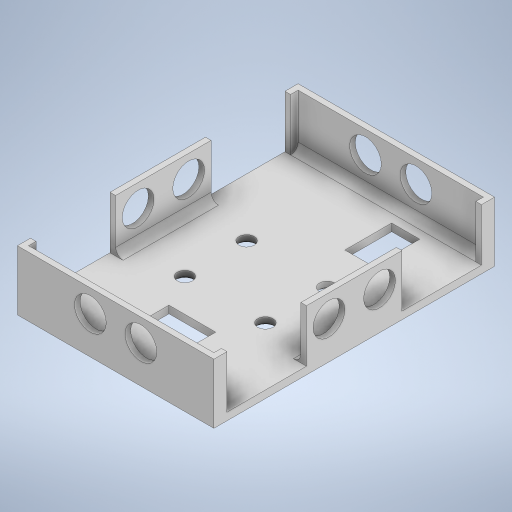
# Autodesk Inventor part: TestingPlatform_base01
Saved by Autodesk Inventor 2024.2 (Build 282272000, 272)
## iProperties
Created: 2024-01-29
Part Number: TestingPlatform_base01
Material: Generic
Document SubType Name: Modeling
Designer: ringl
Density: 1 g/cm^3
Appearance: Default
Author: ringl
Autodesk Inventor part; units mm, degrees
ref_plane "YZ Plane" through (0, 0, 0) normal (1, 0, 0) x (0, 1, 0)
ref_plane "XZ Plane" through (0, 0, 0) normal (0, 1, 0) x (-1, 0, 0)
ref_plane "XY Plane" through (0, 0, 0) normal (0, 0, 1) x (1, 0, 0)
sketch "Sketch1" plane through (0, 0, 0) normal (0, 1, 0) x (-1, 0, 0)
  line L0 (0, 0) -> (58, 0) construction
  line L1 (58, 0) -> (58, -48) construction
  line L2 (58, -48) -> (0, -48) construction
  line L3 (0, -48) -> (0, 0) construction
  circle A0 centre (50.5, -7.5) radius 2.35
  circle A1 centre (50.5, -40.5) radius 2.35
  circle A2 centre (7.5, -7.5) radius 2.35
  circle A3 centre (7.5, -40.5) radius 2.35
  circle A4 centre (50.5, -7.5) radius 5
  circle A5 centre (50.5, -40.5) radius 5
  circle A6 centre (7.5, -7.5) radius 5
  circle A7 centre (7.5, -40.5) radius 5
  dimension "d0" = 58
  dimension "d1" = 48
  dimension "d2" = 4.7
  dimension "d3" = 4.7
  dimension "d4" = 4.7
  dimension "d5" = 4.7
  dimension "d6" = 33
  dimension "d7" = 43
  dimension "d8" = 7.5
  dimension "d9" = 7.5
  dimension "d10" = 7.5
  dimension "d11" = 7.5
  dimension "d12" = 7.5
  dimension "d13" = 7.5
  dimension "d14" = 10
  dimension "d15" = 10
  dimension "d16" = 10
  dimension "d17" = 10
  constraints: 8 centre point, 8 end point, 4 coincident, 2 parallel, 1 horizontal, 1 perpendicular
  measures "d0" distance of L1.end L2.end
  measures "d1" distance of L0.end L1.end
  measures "d2" diameter of A0
  measures "d3" diameter of A1
  measures "d4" diameter of A2
  measures "d5" diameter of A3
  measures "d6" distance of A1.centre A0.centre
  measures "d7" distance of A3.centre A1.centre
  measures "d8" distance from line of L0 A0.centre
  measures "d9" distance from line of L0 A2.centre
  measures "d10" distance from line of L3 A2.centre
  measures "d11" distance from line of L3 A3.centre
  measures "d12" distance from line of L1 A1.centre
  measures "d13" distance from line of L1 A0.centre
  measures "d14" diameter of A4
  measures "d15" diameter of A5
  measures "d16" diameter of A6
  measures "d17" diameter of A7
extrude "Extrusion1" add sketch "Sketch1" along normal blind 12
sketch "Sketch2" plane through (-50.5, 12, -7.5) normal (0, 1, 0) x (1, 0, 0)
  line L0 (-31, -58.5) -> (74, -58.5)
  line L1 (74, -58.5) -> (74, 91.5)
  line L2 (74, 91.5) -> (-31, 91.5)
  line L3 (-31, 91.5) -> (-31, -58.5)
  circle A0 centre (0, 0) radius 2.35 projected
  circle A1 centre (0, 33) radius 2.35 projected
  circle A2 centre (43, 33) radius 2.35 projected
  circle A3 centre (43, 0) radius 2.35 projected
  circle A4 centre (43, 0) radius 2.35
  point P0 (50.5, -7.5)
  dimension "d20" = 105
  dimension "d21" = 150
  dimension "d22" = 58.5
  dimension "d23" = 31
  constraints: 8 end point, 4 coincident, 2 parallel, 1 centre point, 1 horizontal, 1 perpendicular, 1 other
  measures "d20" distance of L2.end L1.end
  measures "d21" distance of L1.end L0.end
  measures "d22" distance from line of L0 point (43, 0)
  measures "d23" distance from line of L3 point (0, 0)
extrude "Extrusion3" add sketch "Sketch2" along normal blind 4
sketch "Sketch3" plane through (-50.5, 16, -7.5) normal (0, 1, 0) x (1, 0, 0)
  line L0 (-31, 91.5) -> (-31, -58.5) projected
  line L1 (-31, -58.5) -> (-31, -38.5)
  line L2 (-31, -38.5) -> (-28, -38.5)
  line L3 (-28, -38.5) -> (-28, -55.5)
  line L4 (-28, -55.5) -> (-11, -55.5)
  line L5 (-11, -58.5) -> (-31, -58.5)
  line L6 (-28, 88.5) -> (-11, 88.5)
  line L7 (74, -58.5) -> (74, 91.5) projected
  line L8 (74, 91.5) -> (54, 91.5)
  line L9 (71, 71.5) -> (74, 71.5)
  line L10 (74, 71.5) -> (74, 91.5)
  line L11 (74, -58.5) -> (74, -38.5)
  line L12 (74, -38.5) -> (71, -38.5)
  line L13 (71, -38.5) -> (71, -55.5)
  line L14 (71, -55.5) -> (54, -55.5)
  line L15 (54, -58.5) -> (74, -58.5)
  line L16 (74, 91.5) -> (-31, 91.5) projected
  line L17 (54, 88.5) -> (71, 88.5)
  line L18 (71, 88.5) -> (71, 71.5)
  line L19 (-11, 91.5) -> (-31, 91.5)
  line L20 (-31, 91.5) -> (-31, 71.5)
  line L21 (-31, 71.5) -> (-28, 71.5)
  line L22 (-28, 71.5) -> (-28, 88.5)
  line L23 (-11, -55.5) -> (54, -55.5)
  line L24 (54, -58.5) -> (-11, -58.5)
  line L25 (-11, 91.5) -> (54, 91.5)
  line L26 (54, 88.5) -> (-11, 88.5)
  point P0 (50.5, -7.5)
  dimension "d28" = 20
  dimension "d48" = 20
  dimension "d49" = 3
  dimension "d50" = 3
  dimension "d51" = 3
  dimension "d52" = 3
  dimension "d53" = 20
  dimension "d55" = 20
  dimension "d56" = 20
  dimension "d57" = 3
  dimension "d69" = 20
  dimension "d95" = 17
  dimension "d96" = 65
  dimension "d102" = 3
  dimension "d103" = 17
  dimension "d104" = 65
  dimension "d105" = 17
  constraints: 48 end point, 10 perpendicular, 6 point on line, 4 collinear, 2 horizontal, 1 parallel
  measures "d28" distance of L0.end L1.end
  measures "d48" distance of L5.start L0.end
  measures "d49" distance of L4.end L5.start
  measures "d50" distance of L1.end L2.end
  measures "d51" distance of L14.end L15.start
  measures "d52" distance of L11.end L12.end
  measures "d53" distance between parallel lines of L15 L12
  measures "d55" distance of L7.end L8.end
  measures "d56" distance of L9.end L7.end
  measures "d57" distance of L9.start L9.end
  measures "d69" distance of L0.start L20.end
  measures "d95" distance of L13.end L14.end
  measures "d96" distance of L4.end L14.end
  measures "d102" distance between parallel lines of L16 L17
  measures "d103" distance of L6.start L6.end
  measures "d104" distance of L17.start L6.end
  measures "d105" distance of L17.start L17.end
extrude "Extrusion4" add sketch "Sketch3" along normal blind 28 contours L16 L8 L7 L9 L18 L17 L26 L6 L22 L21 L0 | L2 L3 L4 L23 L14 L13 L12 L7 L15 L24 L5 L0
sketch "Sketch4" plane through (-81.5, 12, 51) normal (0, 0, 1) x (1, 0, 0)
  line L0 (0, 0) -> (0, 32) projected
  line L1 (0, 0) -> (100, 0)
  line L2 (100, 0) -> (100, -15)
  line L3 (100, -15) -> (0, -15)
  line L4 (0, -15) -> (0, 0)
  point P0 (81.5, -12)
  dimension "d59" = 100
  dimension "d60" = 15
  constraints: 8 end point, 2 parallel, 1 horizontal, 1 perpendicular
  measures "d59" distance of L2.end L3.end
  measures "d60" distance of L1.end L2.end
extrude "remove legs" cut sketch "Sketch4" against normal through all
sketch "Sketch5" plane through (-50.5, 12, -7.5) normal (0, -1, 0) x (1, 0, 0)
  circle A0 centre (0, 0) radius 2.35 projected
  circle A1 centre (0, 0) radius 4.1
  circle A2 centre (43, 0) radius 2.35 projected
  circle A3 centre (43, 0) radius 4.1
  circle A4 centre (43, -33) radius 2.35 projected
  circle A5 centre (43, -33) radius 4.1
  circle A6 centre (0, -33) radius 2.35 projected
  circle A7 centre (0, -33) radius 4.1
  circle A8 centre (0, 0) radius 2.35
  circle A9 centre (43, 0) radius 2.35
  circle A10 centre (43, -33) radius 2.35
  circle A11 centre (0, -33) radius 2.35
  point P0 (50.5, 7.5)
  dimension "d63" = 8.2
  dimension "d64" = 8.2
  dimension "d65" = 8.2
  dimension "d66" = 8.2
  constraints: 8 centre point, 8 coincident, 4 concentric
  measures "d63" diameter of A1
  measures "d64" diameter of A3
  measures "d65" diameter of A5
  measures "d66" diameter of A7
extrude "Extrusion6" cut sketch "Sketch5" against normal blind 4
sketch "Sketch6" plane through (-50.5, 16, -7.5) normal (0, 1, 0) x (1, 0, 0)
  line L0 (9, -17.5) -> (34, -17.5)
  line L1 (34, -17.5) -> (34, -32.5)
  line L2 (34, -32.5) -> (9, -32.5)
  line L3 (9, -32.5) -> (9, -17.5)
  line L4 (30.5, 55) -> (45.5, 55)
  line L5 (45.5, 55) -> (45.5, 80)
  line L6 (45.5, 80) -> (30.5, 80)
  line L7 (30.5, 80) -> (30.5, 55)
  circle A0 centre (43, 33) radius 4.1 construction
  circle A1 centre (0, 33) radius 4.1 construction
  circle A2 centre (0, 0) radius 4.1 construction
  circle A3 centre (43, 0) radius 4.1 construction
  point P0 (50.5, -7.5)
  dimension "d72" = 25
  dimension "d73" = 15
  dimension "d74" = 15
  dimension "d75" = 25
  dimension "d76" = 22
  dimension "d77" = 2.5
  dimension "d78" = 9
  dimension "d79" = 17.5
  constraints: 16 end point, 4 parallel, 2 horizontal, 2 perpendicular
  measures "d72" distance of L0.start L0.end
  measures "d73" distance of L4.start L4.end
  measures "d74" distance of L0.end L1.end
  measures "d75" distance of L4.end L5.end
  measures "d76" distance from line of L4 A0.centre
  measures "d77" distance from line of A0.centre L5
  measures "d78" distance from line of L3 A2.centre
  measures "d79" distance from line of L0 A3.centre
extrude "Extrusion7" cut sketch "Sketch6" against normal blind 10
chamfer "Chamfer1" distance 1 angle 45 4 edges at (-11.6, 12, -7.5) (-11.6, 12, -40.5) (-54.6, 12, -40.5) (-54.6, 12, -7.5)
sketch "Sketch7" plane through (-50.5, 16, -7.5) normal (0, 1, 0) x (1, 0, 0)
  line L0 (74, -38.5) -> (74, 71.5) projected
  line L1 (74, 42) -> (71, 42)
  line L2 (71, 42) -> (71, -9)
  line L3 (71, -9) -> (74, -9)
  line L4 (74, -9) -> (74, 42)
  line L5 (-31, 71.5) -> (-31, -38.5) projected
  line L6 (-31, 42) -> (-28, 42)
  line L7 (-28, 42) -> (-28, -9)
  line L8 (-28, -9) -> (-31, -9)
  line L9 (-31, -9) -> (-31, 42)
  line L10 (-31, -58.5) -> (74, -58.5) projected
  point P0 (50.5, -7.5)
  point P1 (74, -28.5)
  point P2 (74, 61.5)
  point P3 (-31, 67.5)
  point P4 (-31, -28.5)
  point P5 (72.5, 42)
  point P6 (-29.5, 42)
  point P7 (-31, -9)
  point P8 (74, -48.5)
  point P9 (-31, -48.5)
  dimension "d88" = 3
  dimension "d89" = 51
  dimension "d91" = 3
  dimension "d92" = 51
  dimension "d116" = 49.5
  constraints: 16 end point, 4 parallel, 2 horizontal, 2 midpoint, 2 perpendicular, 2 point on line, 1 horizontal alignment
  measures "d88" distance of L1.start L1.end
  measures "d89" distance of L1.end L2.end
  measures "d91" distance of L7.end L8.end
  measures "d92" distance of L6.end L7.end
  measures "d116" distance between parallel lines of L10 L3
sketch "Sketch8" plane through (23.5, 12, 51) normal (1, 0, 0) x (0, 0, -1)
  circle A0 centre (61.5, 20) radius 8.5
  circle A1 centre (88.5, 20) radius 8.5
  line L0 (0, 0) -> (150, 0) projected
  line L1 (0, 0) -> (0, 32) projected
  point P0 (51, -12)
  dimension "d106" = 17
  dimension "d107" = 17
  dimension "d108" = 27
  dimension "d109" = 20
  dimension "d119" = 61.5
  constraints: 2 centre point, 1 horizontal alignment
  measures "d106" diameter of A0
  measures "d107" diameter of A1
  measures "d108" distance of A1.centre A0.centre
  measures "d109" distance from line of L0 A0.centre
  measures "d119" distance from line of L1 A0.centre
sketch "Sketch9" plane through (-81.5, 12, 51) normal (0, 0, 1) x (1, 0, 0)
  circle A0 centre (39, 20) radius 8.5
  circle A1 centre (66, 20) radius 8.5
  line L0 (0, 0) -> (105, 0) projected
  line L1 (0, 0) -> (0, 32) projected
  point P0 (81.5, -12)
  dimension "d113" = 17
  dimension "d114" = 17
  dimension "d115" = 20
  dimension "d124" = 20
  dimension "d125" = 39
  dimension "d126" = 27
  constraints: 2 centre point
  measures "d113" diameter of A0
  measures "d114" diameter of A1
  measures "d115" distance from line of L0 A0.centre
  measures "d124" distance from line of L0 A1.centre
  measures "d125" distance from line of L1 A0.centre
  measures "d126" distance of A1.centre A0.centre
extrude "Extrusion10" add sketch "Sketch7" along normal blind 28
extrude "Extrusion11" cut sketch "Sketch8" against normal through all
extrude "Extrusion12" cut sketch "Sketch9" against normal through all
sketch "Sketch11" plane through (-81.5, 12, -99) normal (-1, 0, 0) x (0, 0, 1)
  line L0 (20, 32) -> (3, 32) projected
  line L1 (3, 4) -> (20, 4) projected
  line L2 (20, 32) -> (7, 32)
  line L3 (7, 32) -> (7, 4)
  line L4 (7, 4) -> (20, 4)
  line L5 (20, 4) -> (20, 32)
  point P0 (99, -12)
  point P1 (20, 4)
  point P2 (7, 32)
  dimension "d127" = 13
  constraints: 8 end point, 2 parallel, 1 horizontal, 1 perpendicular, 1 point on line
  measures "d127" distance between parallel lines of L5 L3
extrude "Extrusion13" cut sketch "Sketch11" against normal through all
fillet "Fillet3" radius 4 2 edges at (20.5, 16, -24) (-78.5, 16, -24)
fillet "Fillet4" radius 4 2 edges at (-29, 16, -96) (-29, 16, 48)
sketch "Sketch12" plane through (-81.5, 12, -99) normal (-1, 0, 0) x (0, 0, 1)
  line L0 (100.5, 4) -> (130, 4) projected
  line L1 (130, 32) -> (150, 32) projected
  line L2 (130, 4) -> (143, 4)
  line L3 (143, 4) -> (143, 32)
  line L4 (143, 32) -> (130, 32)
  line L5 (130, 32) -> (130, 4)
  point P0 (99, -12)
  point P1 (130, 18)
  dimension "d132" = 13
  constraints: 8 end point, 2 parallel, 1 horizontal, 1 midpoint, 1 perpendicular, 1 point on line
  measures "d132" distance from line of point (130, 18) L3
extrude "Extrusion14" cut sketch "Sketch12" against normal through all
body "Solid1"
